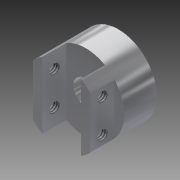
# Autodesk Inventor part: Pneumatic Connector -Actuator Side
Saved by Autodesk Inventor 2013 (Build 170138000, 138)
## iProperties
Created: 2013-06-08
Part Number: Pneumatic Connector -Actuator Side
Material: Generic
Document SubType Name: Modeling
Designer: mvarma
Density: 1 g/cm^3
Author: mvarma
Autodesk Inventor part; units mm, degrees
ref_plane "YZ Plane" through (0, 0, 0) normal (1, 0, 0) x (0, 1, 0)
ref_plane "XZ Plane" through (0, 0, 0) normal (0, 1, 0) x (-1, 0, 0)
sketch "Sketch1" plane through (0, 0, 0) normal (0, 0, 1) x (1, 0, 0)
  arc A0 (-1.508, 2.794) -> (-1.508, -2.794) centre (0, 0) ccw
  line L0 (-3.175, 0) -> (0, 0) construction
  line L1 (0, 0) -> (3.175, 0) construction
  line L2 (-1.508, 2.794) -> (1.508, 2.794)
  line L3 (-1.508, -2.794) -> (1.508, -2.794)
  arc A1 (1.508, 2.794) -> (-1.508, 2.794) centre (0, 0) ccw construction
  arc A2 (1.508, -2.794) -> (1.508, 2.794) centre (0, 0) ccw
  arc A3 (-1.508, -2.794) -> (1.508, -2.794) centre (0, 0) ccw construction
  circle A4 centre (0, 0) radius 3.429 construction
  circle A5 centre (0, 0) radius 4.064
  circle A6 centre (0, 0) radius 12.7
  dimension "d1" = 2.794
  dimension "d2" = 3.175
  dimension "d3" = 6.858
  dimension "d5" = 0.635
  dimension "d6" = 25.4
  constraints: 14 point on circle, 8 end point, 7 centre point, 4 coincident, 2 parallel, 1 collinear, 1 horizontal, 1 other
  measures "d1" distance between parallel lines of L0 L2
  measures "d2" radius of A0
  measures "d3" diameter of A4
  measures "d5" radial gap between concentric circles of A5 A4
  measures "d6" diameter of A6
extrude "Extrusion1" add sketch "Sketch1" along normal blind 3.048 contours A5 | A6
sketch "Sketch2" plane through (0, 0, 3.048) normal (0, 0, 1) x (1, 0, 0)
  circle A0 centre (0, 0) radius 12.7 projected
  arc A1 (-1.508, 2.794) -> (-1.508, -2.794) centre (0, 0) ccw projected
  constraints: 1 coincident
extrude "Extrusion2" add sketch "Sketch2" along normal blind 3.175
hole "Hole1" at (0, 0, 3.048) direction (0, 0, 1) diameter 3.302 depth 25.4 tip angle 118 thread size "8-32 UNC" class "2B" standard "ANSI Unified Screw Threads"
sketch "Sketch3" plane through (0, 0, 6.223) normal (0, 0, 1) x (1, 0, 0)
  circle A0 centre (0, 0) radius 12.7 projected
  circle A1 centre (0, 0) radius 3.429
  circle A2 centre (0, 0) radius 4.064
  dimension "d18" = 6.858
  dimension "d19" = 0.635
  constraints: 2 centre point, 2 coincident
  measures "d18" diameter of A1
  measures "d19" radial gap between concentric circles of A2 A1
extrude "Extrusion3" add sketch "Sketch3" along normal blind 4.572 contours A0
sketch "Sketch4" plane through (0, 0, 10.795) normal (0, 0, 1) x (1, 0, 0)
  circle A0 centre (0, 0) radius 4.064 projected
  circle A1 centre (0, 0) radius 12.7 projected
  line L0 (-6.35, 10.9985) -> (-6.35, -10.9985)
  line L1 (0, 12.7) -> (0, -12.7)
  line L2 (6.35, 10.9985) -> (6.35, -10.9985)
  line L3 (-9.525, 8.4003) -> (-9.525, -8.4003)
  line L4 (9.525, 8.4003) -> (9.525, -8.4003)
  dimension "d22" = 6.35
  dimension "d23" = 3.175
  constraints: 10 end point, 4 parallel, 1 midpoint, 1 vertical, 13 other
  measures "d22" distance between parallel lines of L1 L0
  measures "d23" distance between parallel lines of L0 L3
extrude "Extrusion4" add sketch "Sketch4" along normal blind 7.9375 contours A1 L4 L2 | L0 A1 L3
sketch "Sketch5" plane through (-6.35, -10.9985, 10.795) normal (1, 0, 0) x (0, 0, -1)
  line L0 (0, 21.997) -> (0, 0) projected
  line L1 (0, 21.997) -> (-7.9375, 21.997) projected
  line L2 (-7.9375, 0) -> (-7.9375, 21.997) projected
  line L3 (0, 0) -> (-7.9375, 0) projected
  line L4 (-3.9688, 21.997) -> (-3.9688, 0) construction
  line L5 (-7.9375, 10.9985) -> (0, 10.9985) construction
  line L6 (-7.9375, 16.4978) -> (0, 16.4978) construction
  line L7 (-7.9375, 5.4993) -> (0, 5.4993) construction
  point P0 (10.795, 10.9985)
  point P1 (-3.9688, 16.4978)
  point P2 (-3.9688, 5.4993)
  dimension "d26" = 5.4993
  dimension "d27" = 5.4993
  constraints: 8 end point, 6 midpoint, 4 point on line, 1 parallel, 1 perpendicular, 1 other
  measures "d26" distance between parallel lines of L6 L5
  measures "d27" distance between parallel lines of L1 L6
hole "Hole2" at (-6.35, 5.4993, 14.7638) at (-6.35, -5.4993, 14.7638) direction (-1, 0, 0) diameter 3.302 end through all thread size "8-32 UNC" class "2B" standard "ANSI Unified Screw Threads"
ref_plane "Work Plane1" through (0, -10.9985, 10.795) normal (1, 0, 0) x (0, 0, -1)
mirror "Mirror1" about plane through (0, -10.9985, 10.795) normal (1, 0, 0) of "Hole2"
equation "\"d26\" = d27"
body "Solid1"
